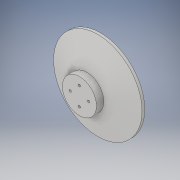
# Autodesk Inventor part: foot
Saved by Autodesk Inventor 2019 (Build 230136000, 136)
## iProperties
Created: 2024-08-06
Part Number: foot
Material: Generisch
Document SubType Name: Modeling
Designer: nic
Density: 1 g/cm^3
Appearance: Vorgabe
Author: nic
Autodesk Inventor part; units mm, degrees
ref_plane "YZ Plane" through (0, 0, 0) normal (1, 0, 0) x (0, 1, 0)
ref_plane "XZ Plane" through (0, 0, 0) normal (0, 1, 0) x (-1, 0, 0)
ref_plane "XY Plane" through (0, 0, 0) normal (0, 0, 1) x (1, 0, 0)
sketch "Skizze1" plane through (0, 0, 0) normal (0, 0, 1) x (1, 0, 0)
  circle A0 centre (0, 0) radius 75
  line L0 (0, 0) -> (13.5, 0) construction
  line L1 (13.5, 0) -> (-13.5, 0) construction
  line L2 (0, 0) -> (0, -13.5) construction
  line L3 (0, -13.5) -> (0, 13.5) construction
  circle A1 centre (0, 13.5) radius 1.6
  circle A2 centre (13.5, 0) radius 1.6
  circle A3 centre (0, -13.5) radius 1.6
  circle A4 centre (-13.5, 0) radius 1.6
  dimension "d0" = 150
  dimension "d1" = 13.5
  dimension "d2" = 27
  dimension "d3" = 13.5
  dimension "d4" = 27
  dimension "d5" = 3.2
  dimension "d6" = 3.2
  dimension "d7" = 3.2
  dimension "d8" = 3.2
  constraints: 8 end point, 5 centre point, 5 coincident, 2 point on line, 1 horizontal, 1 vertical
  measures "d0" diameter of A0
  measures "d1" distance of L0.start L0.end
  measures "d2" distance of L0.end L1.end
  measures "d3" distance of L0.start L2.end
  measures "d4" distance of L2.end L3.end
  measures "d5" diameter of A1
  measures "d6" diameter of A2
  measures "d7" diameter of A3
  measures "d8" diameter of A4
extrude "Extrusion1" add sketch "Skizze1" along normal blind 21
sketch "Skizze2" plane through (0, 0, 0) normal (0, 0, -1) x (-1, 0, 0)
  circle A0 centre (13.5, 0) radius 1.6 projected
  circle A1 centre (0, -13.5) radius 1.6 projected
  circle A2 centre (-13.5, 0) radius 1.6 projected
  circle A3 centre (0, 13.5) radius 1.6 projected
  circle A4 centre (0, 0) radius 75 projected
  circle A5 centre (13.5, 0) radius 1.6 projected
  line L0 (16, 2.5) -> (11, 2.5)
  line L1 (11, 2.5) -> (11, -2.5)
  line L2 (11, -2.5) -> (16, -2.5)
  line L3 (16, -2.5) -> (16, 2.5)
  line L4 (16, 2.5) -> (11, -2.5) construction
  line L5 (11, 2.5) -> (16, -2.5) construction
  line L6 (2.5, 16) -> (-2.5, 16)
  line L7 (-2.5, 16) -> (-2.5, 11)
  line L8 (-2.5, 11) -> (2.5, 11)
  line L9 (2.5, 11) -> (2.5, 16)
  line L10 (2.5, 16) -> (-2.5, 11) construction
  line L11 (-2.5, 16) -> (2.5, 11) construction
  line L12 (-11, 2.5) -> (-16, 2.5)
  line L13 (-16, 2.5) -> (-16, -2.5)
  line L14 (-16, -2.5) -> (-11, -2.5)
  line L15 (-11, -2.5) -> (-11, 2.5)
  line L16 (-11, 2.5) -> (-16, -2.5) construction
  line L17 (-16, 2.5) -> (-11, -2.5) construction
  line L18 (2.5, -11) -> (-2.5, -11)
  line L19 (-2.5, -11) -> (-2.5, -16)
  line L20 (-2.5, -16) -> (2.5, -16)
  line L21 (2.5, -16) -> (2.5, -11)
  line L22 (2.5, -11) -> (-2.5, -16) construction
  line L23 (-2.5, -11) -> (2.5, -16) construction
  dimension "d11" = 5
  dimension "d12" = 5
  dimension "d13" = 5
  dimension "d14" = 5
  dimension "d15" = 5
  dimension "d16" = 5
  dimension "d17" = 5
  dimension "d18" = 5
  constraints: 48 end point, 8 midpoint, 8 parallel, 4 horizontal, 4 perpendicular
  measures "d11" distance of L2.end L1.end
  measures "d12" distance of L1.end L0.end
  measures "d13" distance of L8.end L7.end
  measures "d14" distance of L7.end L6.end
  measures "d15" distance of L14.end L13.end
  measures "d16" distance of L13.end L12.end
  measures "d17" distance of L20.end L19.end
  measures "d18" distance of L19.end L18.end
extrude "Extrusion2" cut sketch "Skizze2" against normal blind 4 contours L3 L2 L1 L0 | L9 L8 L7 L6 | L15 L14 L13 L12 | L21 L20 L19 L18
draft "Flächenverjüngung1" angle -68 pull direction (0, 0, -1) faces at (-33.9595, -66.8711, 14) fixed edges at (-75, 0, 0)
sketch "Skizze3" plane through (0, 0, 21) normal (0, 0, 1) x (1, 0, 0)
  circle A0 centre (0, 0) radius 75 projected
  circle A1 centre (0, 0) radius 65
  dimension "d22" = 10
  constraints: 1 centre point
  measures "d22" radial gap between concentric circles of A0 A1
extrude "Extrusion3" cut sketch "Skizze3" against normal through all
sketch "Skizze4" plane through (0, 0, 21) normal (0, 0, 1) x (1, 0, 0)
  circle A0 centre (0, 0) radius 25
  circle A1 centre (-13.5, 0) radius 1.6 projected
  circle A2 centre (0, -13.5) radius 1.6 projected
  circle A3 centre (13.5, 0) radius 1.6 projected
  circle A4 centre (0, 13.5) radius 1.6 projected
  dimension "d25" = 50
  constraints: 1 centre point, 1 coincident
  measures "d25" diameter of A0
extrude "Extrusion4" add sketch "Skizze4" against normal blind 5
sketch "Skizze5" plane through (0, 0, 21) normal (0, 0, 1) x (1, 0, 0)
  circle A0 centre (0, 0) radius 25 projected
  circle A1 centre (-13.5, 0) radius 1.6 projected
  circle A2 centre (0, -13.5) radius 1.6 projected
  circle A3 centre (13.5, 0) radius 1.6 projected
  circle A4 centre (0, 13.5) radius 1.6 projected
extrude "Extrusion5" add sketch "Skizze5" along normal blind 10
sketch "Skizze6" plane through (0, 0, 0) normal (0, 0, -1) x (-1, 0, 0)
  line L0 (16.5, -16.5) -> (-16.5, -16.5)
  line L1 (-16.5, -16.5) -> (-16.5, 16.5)
  line L2 (-16.5, 16.5) -> (16.5, 16.5)
  line L3 (16.5, 16.5) -> (16.5, -16.5)
  line L4 (16.5, -16.5) -> (-16.5, 16.5) construction
  line L5 (-16.5, -16.5) -> (16.5, 16.5) construction
  point P0 (0, 0)
  dimension "d30" = 33
  dimension "d31" = 33
  constraints: 12 end point, 2 midpoint, 2 parallel, 1 horizontal, 1 perpendicular
  measures "d30" distance of L1.end L2.end
  measures "d31" distance of L0.end L1.end
extrude "Extrusion6" cut sketch "Skizze6" against normal blind 11
